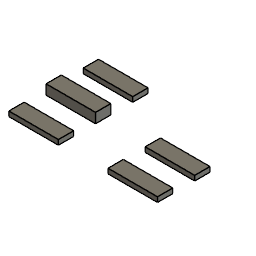
Button(s) ignore the tiny ones idk how to export just one button to f3d (Autodesk Fusion 360 design; units mm, degrees)
Autodesk Fusion 360 part; units mm, degrees
note: some values were not read from the file. Set by a fixed rule: which sketch regions a step uses.
sketch "Sketch1" plane through (0, 0, 0) normal (0, 1, 0) x (1, 0, 0)
  line L0 (-19, 5) -> (1, 5)
  line L1 (1, 5) -> (1, -1.2)
  line L2 (1, -1.2) -> (-19, -1.2)
  line L3 (-19, -1.2) -> (-19, 5)
  dimension "d1" = 20
  dimension "d2" = 6.2
  constraint horizontal L0
  constraint vertical L1
  constraint horizontal L2
  constraint vertical L3
  measures "d1" distance of L0.start L0.end
  measures "d2" distance of L0.end L1.end
extrude "Extrude1" add sketch "Sketch1" along normal blind 2 makes body 1
copy_body "CopyPasteBodies1" bodies 1 makes body 2
move_body "Move1" bodies 2 to x (1, 0, 0) y (0, 1, 0) z (0, 0, 1) at (40, 0, 0)
copy_body "CopyPasteBodies2" bodies 2 makes body 3
move_body "Move2" bodies 3 to x (1, 0, 0) y (0, 1, 0) z (0, 0, 1) at (0, 0, 15)
copy_body "CopyPasteBodies3" bodies 2 makes body 4
move_body "Move3" bodies 4 to x (1, 0, 0) y (0, 1, 0) z (0, 0, 1) at (40, 0, 0)
copy_body "CopyPasteBodies4" bodies 2 makes body 5
move_body "Move4" bodies 5 to x (1, 0, 0) y (0, 1, 0) z (0, 0, 1) at (40, 0, 15)
move_body "Move5" bodies 1 to x (1, 0, 0) y (0, 1, 0) z (0, 0, 1) at (40, 0, -15)
sketch "Sketch2" plane through (0, 2, 0) normal (0, 1, 0) x (-1, 0, 0)
  line L0 (-61, 1.2) -> (-81, 1.2)
  line L1 (-81, 1.2) -> (-81, -5)
  line L2 (-81, -5) -> (-61, -5)
  line L3 (-61, -5) -> (-61, 1.2)
  line L4 (-73.1233, -3.6071) -> (-73.1233, 0.3967) construction
  line L5 (-77.7702, -1.6052) -> (-68.4763, -1.6052) construction
sketch "Sketch3" plane through (0, 2, 0) normal (0, 1, 0) x (-1, 0, 0)
  line L0 (-61, 16.2) -> (-81, 16.2)
  line L1 (-81, 16.2) -> (-81, 10)
  line L2 (-81, 10) -> (-61, 10)
  line L3 (-61, 10) -> (-61, 16.2)
  line L4 (-67.2606, 15.7358) -> (-76.5545, 15.7358) construction
  line L5 (-76.5545, 15.7358) -> (-76.5545, 11.732) construction
  line L6 (-76.5545, 11.732) -> (-67.2606, 11.732) construction
  line L7 (-67.2606, 11.732) -> (-67.2606, 15.7358) construction
  line L8 (-22.292, 0.7745) -> (-46.644, 0.7399) construction
  line L9 (-46.644, 0.7399) -> (-46.6383, -3.2647) construction
  line L10 (-46.6383, -3.2647) -> (-22.2863, -3.2301) construction
  line L11 (-22.2863, -3.2301) -> (-22.292, 0.7745) construction
  line L12 (-22.4171, -14.6783) -> (-44.6811, -14.6634) construction
  line L13 (-44.6811, -14.6634) -> (-44.6837, -18.6672) construction
  line L14 (-44.6837, -18.6672) -> (-22.4197, -18.682) construction
  line L15 (-22.4197, -18.682) -> (-22.4171, -14.6783) construction
  line L16 (-22.8704, 15.3217) -> (-47.6774, 15.3266) construction
  line L17 (-47.6774, 15.3266) -> (-47.6781, 11.3229) construction
  line L18 (-47.6781, 11.3229) -> (-22.8712, 11.318) construction
  line L19 (-22.8712, 11.318) -> (-22.8704, 15.3217) construction
  dimension "d6" = 3
  dimension "d7" = 2.5
  dimension "d8" = 3
  dimension "d9" = 2.5
sketch "Sketch4" plane through (0, 0, 0) normal (0, -1, 0) x (1, 0, 0)
  line L0 (41, -13.8) -> (21, -13.8)
  line L1 (21, -13.8) -> (21, -20)
  line L2 (21, -20) -> (41, -20)
  line L3 (41, -20) -> (41, -13.8)
  circle A0 centre (32, -17) radius 2.05
  dimension "d12" = 4.1
  measures "d12" diameter of A0
extrude "Extrude3" cut sketch "Sketch4" against normal blind 0.5 contours A0 bodies 1
extrude "Extrude4" cut 1 faces at (32.595, 0.5, -16.4136) along direction (0, 1, 0) blind 0.5 on bodies 1 bodies 1
sketch "Sketch5" plane through (0, 0, 0) normal (0, -1, 0) x (1, 0, 0)
  line L0 (41, 1.2) -> (21, 1.2)
  line L1 (21, 1.2) -> (21, -5)
  line L2 (21, -5) -> (41, -5)
  line L3 (41, -5) -> (41, 1.2)
  circle A0 centre (31, -1.9) radius 2
sketch "Sketch6" plane through (0, 0, 0) normal (0, -1, 0) x (1, 0, 0)
  line L0 (81, 1.2) -> (61, 1.2)
  line L1 (61, 1.2) -> (61, -5)
  line L2 (61, -5) -> (81, -5)
  line L3 (81, -5) -> (81, 1.2)
  circle A0 centre (73, -1.9) radius 2
  circle A1 centre (73, 13) radius 2
  dimension "d19" = 4
  dimension "d20" = 4
  measures "d19" diameter of A0
  measures "d20" diameter of A1
extrude "Extrude5" cut sketch "Sketch5" sketch "Sketch6" against normal blind 1 contours A0 of sketch 2 contours A0 | A1 bodies 2 3 4 5
extrude "Extrude6" add 1 faces at (27.6667, 2, -2.9333) along direction (0, 1, 0) blind 2 on bodies 2 bodies 2
extrude "Extrude7" add 1 faces at (31.3037, 1, -2.1215) along direction (0, -1, 0) blind 0.1 on bodies 2 bodies 2
equation "d17 = 'Start Passive'"
equation "d18 = 'End Passive'"
named bodies: "Clock Set"
